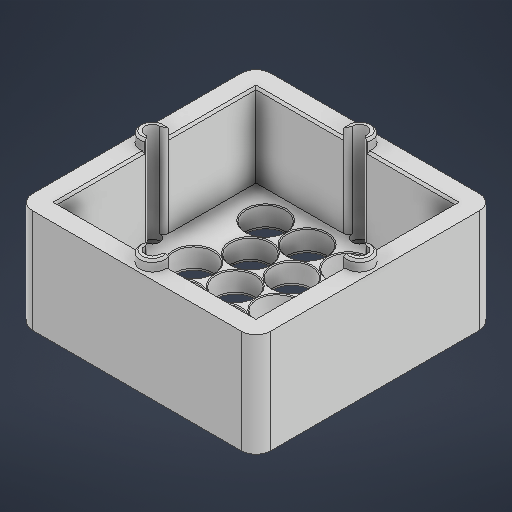
# Autodesk Inventor part: Battery Holder (Top)
Saved by Autodesk Inventor 2025 (Build 290162000, 162)
## iProperties
Created: 2025-08-08
Part Number: Battery Holder (Top)
Material: Generic
Document SubType Name: Modeling
Designer: mayhe
Density: 1 g/cm^3
Appearance: Default
Author: mayhe
Autodesk Inventor part; units mm, degrees
ref_plane "YZ Plane" through (0, 0, 0) normal (1, 0, 0) x (0, 1, 0)
ref_plane "XZ Plane" through (0, 0, 0) normal (0, 1, 0) x (-1, 0, 0)
ref_plane "XY Plane" through (0, 0, 0) normal (0, 0, 1) x (1, 0, 0)
sketch "Sketch1" plane through (0, 0, 0) normal (0, 1, 0) x (-1, 0, 0)
  line L0 (57.5, 57.5) -> (-57.5, 57.5)
  line L1 (-57.5, 57.5) -> (-57.5, -57.5)
  line L2 (-57.5, -57.5) -> (57.5, -57.5)
  line L3 (57.5, -57.5) -> (57.5, 57.5)
  line L4 (57.5, 57.5) -> (-57.5, -57.5) construction
  line L5 (-57.5, 57.5) -> (57.5, -57.5) construction
  point P0 (0, 0)
  dimension "d0" = 115
  dimension "d1" = 115
  constraints: 12 end point, 2 midpoint, 2 parallel, 1 horizontal, 1 perpendicular
  measures "d0" distance of L2.end L1.end
  measures "d1" distance of L1.end L0.end
extrude "Extrusion1" add sketch "Sketch1" along normal blind 10
sketch "Sketch4" plane through (0, 10, 0) normal (0, 1, 0) x (1, 0, 0)
  line L0 (-48, -48) -> (48, -48)
  line L1 (48, -48) -> (48, 48)
  line L2 (48, 48) -> (-48, 48)
  line L3 (-48, 48) -> (-48, -48)
  line L4 (-57.5, 57.5) -> (-57.5, -57.5) projected
  line L5 (-57.5, 0) -> (-48, 0)
  line L6 (-30, 34.641) -> (30, -34.641) construction
  line L7 (30, 34.641) -> (-30, -34.641) construction
  circle A0 centre (-30, 34.641) radius 9.5
  circle A1 centre (-10, 34.641) radius 9.5
  circle A2 centre (10, 34.641) radius 9.5
  circle A3 centre (30, 34.641) radius 9.5
  circle A4 centre (-30, 0) radius 9.5
  circle A5 centre (-10, 0) radius 9.5
  circle A6 centre (10, 0) radius 9.5
  circle A7 centre (30, 0) radius 9.5
  circle A8 centre (-30, -34.641) radius 9.5
  circle A9 centre (-10, -34.641) radius 9.5
  circle A10 centre (10, -34.641) radius 9.5
  circle A11 centre (30, -34.641) radius 9.5
  circle A12 centre (-20, 17.3205) radius 9.5
  circle A13 centre (0, 17.3205) radius 9.5
  circle A14 centre (20, 17.3205) radius 9.5
  circle A15 centre (-20, -17.3205) radius 9.5
  circle A16 centre (0, -17.3205) radius 9.5
  circle A17 centre (20, -17.3205) radius 9.5
  line L8 (-57.5, -57.5) -> (57.5, -57.5) projected
  line L9 (-57.5, 57.5) -> (57.5, 57.5)
  line L10 (57.5, 57.5) -> (57.5, -57.5)
  line L11 (57.5, -57.5) -> (-57.5, -57.5)
  line L12 (-57.5, -57.5) -> (-57.5, 57.5)
  point P0 (47.3285, -94.6135)
  point P1 (-53.5957, 219.1108)
  point P2 (0, 0)
  point P3 (48, 0)
  point P4 (0, -48)
  point P5 (0, -57.5)
  dimension "d0" = 115
  dimension "d1" = 115
  dimension "d48" = 96
  dimension "d49" = 96
  dimension "d132" = 60
  dimension "d133" = 69.282
  dimension "d134" = 19
  dimension "d137" = 20
  dimension "d140" = 34.641
  dimension "d143" = 19
  dimension "d146" = 10
  dimension "d147" = 17.3205
  dimension "d150" = 20
  dimension "d153" = 34.641
  constraints: 22 end point, 18 centre point, 8 midpoint, 4 horizontal, 4 parallel, 2 perpendicular, 2 vertical, 1 coincident, 1 horizontal alignment, 1 vertical alignment, 32 other
  measures "d48" distance of L2.end L1.end
  measures "d49" distance of L1.end L0.end
  measures "d132" distance of L6.end L7.end
  measures "d133" distance of L7.start L6.end
  measures "d134" diameter of A0
  measures "d137" distance of A0.centre A1.centre
  measures "d140" distance of A0.centre A4.centre
  measures "d143" diameter of A12
  measures "d146" horizontal distance of A1.centre A12.centre
  measures "d147" vertical distance of A12.centre A1.centre
  measures "d150" distance of A12.centre A13.centre
  measures "d153" distance of A12.centre A15.centre
extrude "Extrusion3" add sketch "Sketch4" along normal blind 40 contours L9 L10 L8 L4
hole "Hole4" at (-30, 10, -34.641) at (-10, 10, -34.641) at (10, 10, -34.641) at (30, 10, -34.641) at (20, 10, -17.3205) at (0, 10, -17.3205) at (-20, 10, -17.3205) at (-30, 10, 0) at (-10, 10, 0) at (10, 10, 0) at (30, 10, 0) at (-20, 10, 17.3205) at (0, 10, 17.3205) at (20, 10, 17.3205) at (-30, 10, 34.641) at (-10, 10, 34.641) at (10, 10, 34.641) at (30, 10, 34.641) direction (0, -1, 0) diameter 18.6 end through all countersink diameter 19 countersink angle 2.5
sketch "Sketch6" plane through (0, 0, 0) normal (0, -1, 0) x (1, 0, 0)
  line L0 (50, 50) -> (-50, 50)
  line L1 (-50, 50) -> (-50, -50)
  line L2 (-50, -50) -> (50, -50)
  line L3 (50, -50) -> (50, 50)
  line L4 (50, 50) -> (-50, -50) construction
  line L5 (-50, 50) -> (50, -50) construction
  circle A0 centre (-50, -50) radius 3
  circle A1 centre (0, -50) radius 3
  circle A2 centre (50, -50) radius 3
  circle A3 centre (-50, 0) radius 3
  circle A4 centre (0, 0) radius 3
  circle A5 centre (50, 0) radius 3
  circle A6 centre (-50, 50) radius 3
  circle A7 centre (0, 50) radius 3
  circle A8 centre (50, 50) radius 3
  dimension "d183" = 100
  dimension "d184" = 100
  dimension "d185" = 6
  dimension "d188" = 50
  dimension "d191" = 50
  constraints: 12 end point, 9 centre point, 2 horizontal, 2 midpoint, 2 parallel, 1 coincident, 1 perpendicular, 1 vertical, 16 other
  measures "d183" distance of L2.end L1.end
  measures "d184" distance of L1.end L0.end
  measures "d185" diameter of A0
  measures "d188" distance of A0.centre A1.centre
  measures "d191" distance of A0.centre A3.centre
hole "Hole5" at (-50, 0, 0) at (0, 0, -50) at (50, 0, 0) at (0, 0, 50) direction (0, 1, 0) diameter 7.125 end through all counterbore diameter 13 counterbore depth 7
sketch "Sketch7" plane through (0, 50, 0) normal (0, 1, 0) x (1, 0, 0)
  arc A0 (-48, 2.9481) -> (-48, -2.9481) centre (-50, 0) ccw projected
  arc A1 (-48, 5.6569) -> (-48, -5.6569) centre (-50, 0) ccw
  circle A2 centre (50, 0) radius 6.5 projected
  arc A3 (48, -5.6569) -> (48, 5.6569) centre (50, 0) ccw
  circle A4 centre (0, 50) radius 3.5625 projected
  arc A5 (5.6569, 48) -> (-5.6569, 48) centre (0, 50) ccw
  arc A6 (-2.9481, -48) -> (2.9481, -48) centre (0, -50) ccw projected
  arc A7 (-5.6569, -48) -> (5.6569, -48) centre (0, -50) ccw
  line L0 (-2.9481, 48) -> (-48, 48) projected
  line L1 (48, -48) -> (2.9481, -48) projected
  line L2 (-48, 48) -> (48, 48)
  line L3 (48, 48) -> (48, -48)
  line L4 (48, -48) -> (-48, -48)
  line L5 (-48, -48) -> (-48, 48)
  arc A8 (-48, 2.9481) -> (-48, -2.9481) centre (-50, 0) ccw
  arc A9 (-2.9481, -48) -> (2.9481, -48) centre (0, -50) ccw
  arc A10 (48, -2.9481) -> (48, 2.9481) centre (50, 0) ccw
  arc A11 (2.9481, 48) -> (-2.9481, 48) centre (0, 50) ccw
  point P0 (0, 0)
  point P1 (-48, 2.9481)
  point P2 (-48, -2.9481)
  point P3 (-2.9481, -48)
  point P4 (5.6569, -48)
  point P5 (-5.6569, 48)
  dimension "d201" = 12
  dimension "d202" = 12
  dimension "d203" = 12
  dimension "d204" = 12
  constraints: 16 point on circle, 16 point on line, 8 centre point, 8 coincident, 8 end point, 2 concentric, 2 parallel, 1 horizontal, 1 perpendicular, 2 other
  measures "d201" diameter of A1
  measures "d202" diameter of A3
  measures "d203" diameter of A5
  measures "d204" diameter of A7
extrude "Extrusion4" add sketch "Sketch7" along normal blind 5 contours A0 L5 A1 | A5 L2 A4 L0 | L4 A6 L1 A7 | A3 L3 A10
fillet "Fillet1" radius 7.125 4 edges at (-57.5, 25, -57.5) (57.5, 25, -57.5) (57.5, 25, 57.5) (-57.5, 25, 57.5)
fillet "Fillet2" radius 2 16 edges at (-2.9481, 52.5, -48) (-2.9481, 30, -48) (2.9481, 30, -48) (2.9481, 52.5, -48) (48, 52.5, -2.9481) (48, 30, -2.9481) (48, 30, 2.9481) (48, 52.5, 2.9481) (2.9481, 52.5, 48) (2.9481, 30, 48) (-2.9481, 30, 48) (-2.9481, 52.5, 48) (-48, 52.5, 2.9481) (-48, 30, 2.9481) (-48, 30, -2.9481) (-48, 52.5, -2.9481)
chamfer "Chamfer1" distance 0.4 angle 45 18 edges at (-30, 10, -9.5) (-20, 10, 7.8205) (-10, 10, -9.5) (-30, 10, 25.141) (-10, 10, 25.141) (10, 10, 25.141) (30, 10, 25.141) (20, 10, 7.8205) (0, 10, 7.8205) (10, 10, -9.5) (30, 10, -9.5) (20, 10, -26.8205) (0, 10, -26.8205) (-20, 10, -26.8205) (30, 10, -44.141) (10, 10, -44.141) (-10, 10, -44.141) (-30, 10, -44.141)
chamfer "Chamfer2" distance 1 angle 45 12 edges at (0, 55, -56) (-56, 55, 0) (0, 55, 56) (56, 55, 0) (-26.8284, 50, -48) (-48, 50, -26.8284) (48, 50, -26.8284) (26.8284, 50, -48) (48, 50, 26.8284) (26.8284, 50, 48) (-26.8284, 50, 48) (-48, 50, 26.8284)
equation "\"d153\" = d124"
equation "\"d124\" = 34.641016"
body "Solid1"
